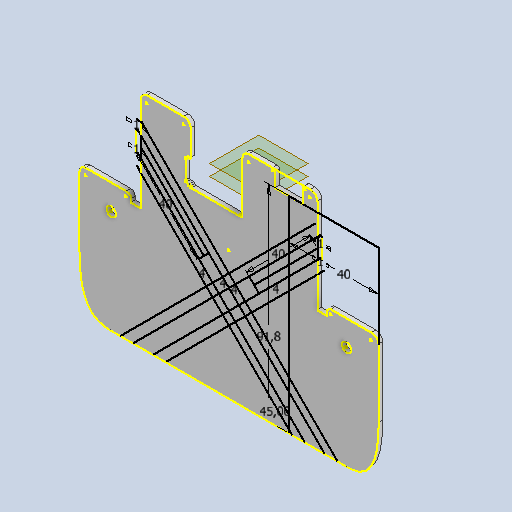
# Autodesk Inventor part: commutationCATboard
Saved by Autodesk Inventor 2022 (Build 260153000, 153)
## iProperties
Created: 2024-07-28
Part Number: commutationCATboard
Material: Типовые
Document SubType Name: Modeling
Designer: Капустяник Андрей
Density: 1 g/cm^3
Appearance: По умолчанию
Author: Капустяник Андрей
Autodesk Inventor part; units mm, degrees
ref_plane "YZ Plane" through (0, 0, 0) normal (1, 0, 0) x (0, 1, 0)
ref_plane "XZ Plane" through (0, 0, 0) normal (0, 1, 0) x (-1, 0, 0)
ref_plane "XY Plane" through (0, 0, 0) normal (0, 0, 1) x (1, 0, 0)
sketch "Эскиз1" plane through (0, 0, 0) normal (0, 0, 1) x (1, 0, 0)
  line L0 (40.5, 52.5) -> (-40.5, 52.5)
  line L1 (-40.5, 52.5) -> (-40.5, -52.5)
  line L2 (-40.5, -52.5) -> (40.5, -52.5)
  line L3 (40.5, -52.5) -> (40.5, 52.5)
  line L4 (40.5, 52.5) -> (-40.5, -52.5) construction
  line L5 (-40.5, 52.5) -> (40.5, -52.5) construction
  line L6 (-14, 32.35) -> (-14, 10.65) projected
  line L7 (-19.5, 32.35) -> (-14, 32.35) projected
  line L8 (-19.5, 10.65) -> (-19.5, 32.35) projected
  line L9 (-14, 10.65) -> (-19.5, 10.65) projected
  line L10 (43.5, -38.5) -> (43.5, -0.445) projected
  line L11 (43.5, 81.5) -> (62.7947, 81.5) projected
  line L12 (62.7947, 81.5) -> (62.7947, -38.5) projected
  line L13 (62.7947, -38.5) -> (43.5, -38.5) projected
  line L14 (-43.5, 81.5) -> (-43.5, 44.5704) projected
  line L15 (-43.5, -38.5) -> (-62.7947, -38.5) projected
  line L16 (-62.7947, -38.5) -> (-62.7947, 81.5) projected
  line L17 (-62.7947, 81.5) -> (-43.5, 81.5) projected
  line L18 (5, 81.5) -> (-5, 81.5) projected
  line L19 (-5, 81.5) -> (-5, 100.5) projected
  line L20 (-5, 100.5) -> (-52.7636, 100.5) projected
  spline S0 degree 4 poles (-64.1096, 93.28) (-61.9791, 96.5946) (-57.9302, 99.8171) (-55.7161, 100.5) (-52.7636, 100.5) knots 0 0 0 0 0 1 1 1 1 1 projected
  spline S1 degree 2 poles (-66.7947, 76.5) (-67.1982, 88.4748) (-64.1096, 93.28) knots 0 0 0 0.595731 0.595731 0.595731 projected
  line L21 (-66.7947, -33.5) -> (-66.7947, 76.5) projected
  spline S2 degree 2 poles (-66.7947, -33.5) (-67.1982, -45.4748) (-64.1096, -50.28) knots 0 0 0 0.595731 0.595731 0.595731 projected
  spline S3 degree 4 poles (-64.1096, -50.28) (-64.1007, -50.2939) (-64.0918, -50.3077) (-64.0828, -50.3215) (-64.0738, -50.3354) knots 0 0 0 0 0 0.004174 0.004174 0.004174 0.004174 0.004174 projected
  spline S4 degree 4 poles (-63.2279, -51.5022) (-63.4539, -51.2466) (-63.6704, -50.967) (-63.8771, -50.6631) (-64.0738, -50.3354) knots -0.674888 -0.674888 -0.674888 -0.674888 -0.674888 -0.60128 -0.60128 -0.60128 -0.60128 -0.60128 projected
  spline S5 degree 4 poles (-63.2279, -51.5022) (-60.8937, -54.4302) (-57.5114, -56.9383) (-55.4411, -57.5) (-52.7636, -57.5) knots 0.093114 0.093114 0.093114 0.093114 0.093114 1 1 1 1 1 projected
  line L22 (-6, -57.5) -> (-52.7636, -57.5) projected
  line L23 (-6, -57.5) -> (-6, -41.6467) projected
  arc A0 (-5, -40.6467) -> (-6, -41.6467) centre (-5, -41.6467) ccw projected
  line L24 (-5, -40.6467) -> (5, -40.6467) projected
  arc A1 (6, -41.6467) -> (5, -40.6467) centre (5, -41.6467) ccw projected
  line L25 (6, -41.6467) -> (6, -57.5) projected
  line L26 (52.7636, -57.5) -> (6, -57.5) projected
  spline S6 degree 4 poles (64.1096, -50.28) (61.9791, -53.5946) (57.9302, -56.8171) (55.7161, -57.5) (52.7636, -57.5) knots 0 0 0 0 0 1 1 1 1 1 projected
  spline S7 degree 2 poles (66.7947, -33.5) (67.1982, -45.4748) (64.1096, -50.28) knots 0 0 0 0.595731 0.595731 0.595731 projected
  line L27 (66.7947, 76.5) -> (66.7947, -33.5) projected
  spline S8 degree 2 poles (64.1096, 93.28) (67.1982, 88.4748) (66.7947, 76.5) knots -0.595731 -0.595731 -0.595731 0 0 0 projected
  spline S9 degree 4 poles (64.1096, 93.28) (61.9791, 96.5946) (57.9302, 99.8171) (55.7161, 100.5) (52.7636, 100.5) knots 0 0 0 0 0 1 1 1 1 1 projected
  line L28 (52.7636, 100.5) -> (5, 100.5) projected
  line L29 (5, 100.5) -> (5, 81.5) projected
  line L30 (33.1, -39.1) -> (40.1, -39.1) projected
  line L31 (40.1, -39.1) -> (40.1, -53.2) projected
  line L32 (40.1, -53.2) -> (33.1, -53.2) projected
  line L33 (33.1, -53.2) -> (33.1, -39.1) projected
  line L34 (-40.1, -39.25) -> (-33.1, -39.25) projected
  line L35 (-33.1, -39.25) -> (-33.1, -53.2) projected
  line L36 (-33.1, -53.2) -> (-40.1, -53.2) projected
  line L37 (-40.1, -53.2) -> (-40.1, -39.25) projected
  line L38 (-3.8, 71.4698) -> (15.7, 71.4698) projected
  arc A2 (18.7, 68.4698) -> (15.7, 71.4698) centre (15.7, 68.4698) ccw projected
  line L39 (18.7, 68.4698) -> (18.7, 55.2061) projected
  arc A3 (15.7, 52.2061) -> (18.7, 55.2061) centre (15.7, 55.2061) ccw projected
  line L40 (15.7, 52.2061) -> (-3.8, 52.2061) projected
  arc A4 (-6.8, 55.2061) -> (-3.8, 52.2061) centre (-3.8, 55.2061) ccw projected
  line L41 (-6.8, 55.2061) -> (-6.8, 68.4698) projected
  arc A5 (-3.8, 71.4698) -> (-6.8, 68.4698) centre (-3.8, 68.4698) ccw projected
  line L42 (40.5, -14.6467) -> (40.5, -35.25) projected
  line L43 (40.5, -35.25) -> (25.5, -35.25) projected
  line L44 (27.6138, 43.5704) -> (40, 43.5704) projected
  line L45 (-27.6138, 43.5704) -> (-27.6138, 44.6963) projected
  line L46 (-27.6138, 44.6963) -> (-10.238, 44.6963) projected
  line L47 (-10.238, 44.6963) -> (-10.238, 43.5704) projected
  line L48 (-10.238, 43.5704) -> (-5, 43.5704) projected
  line L49 (-5, 43.5704) -> (-5, 46.5704) projected
  line L50 (-5, 46.5704) -> (5, 46.5704) projected
  line L51 (5, 46.5704) -> (5, 43.5704) projected
  line L52 (10.238, 43.5704) -> (10.238, 44.6963) projected
  line L53 (10.238, 44.6963) -> (27.6138, 44.6963) projected
  line L54 (27.6138, 44.6963) -> (27.6138, 43.5704) projected
  line L55 (5, 43.5704) -> (10.238, 43.5704) projected
  line L56 (-43.5, 41.5) -> (43.5, 41.5)
  line L57 (43.5, 41.5) -> (43.5, -57.5)
  line L58 (43.5, -57.5) -> (-43.5, -57.5)
  line L59 (-43.5, -57.5) -> (-43.5, 41.5)
  line L60 (40, 41.5) -> (-40, 41.5) projected
  line L61 (25.5, -35.25) -> (25.5, -14.6467) projected
  line L62 (25.5, -14.6467) -> (40.5, -14.6467) projected
  line L63 (-40, 43.5704) -> (-27.6138, 43.5704) projected
  line L64 (43.5, 44.5704) -> (43.5, 81.5) projected
  line L65 (43.5, -0.445) -> (-43.5, -0.445) projected
  line L66 (-43.5, -0.445) -> (-43.5, -38.5) projected
  line L67 (40, 44.5704) -> (43.5, 44.5704) projected
  line L68 (-43.5, 44.5704) -> (-40, 44.5704) projected
  line L69 (-40, 44.5704) -> (-40, 43.5704) projected
  line L70 (40, 43.5704) -> (40, 44.5704) projected
  circle A6 centre (33.954, 52.6704) radius 1.5 projected
  circle A7 centre (23.0046, 73.1714) radius 1.5 projected
  circle A8 centre (-23.0046, 73.1714) radius 1.5 projected
  circle A9 centre (-33.954, 52.6704) radius 1.5 projected
  circle A10 centre (35.5, -5.945) radius 1.25 projected
  circle A11 centre (-35.5, -5.945) radius 1.25 projected
  point P0 (0, 0)
  point P1 (-40.5, 41.35)
  point P2 (40.5, 41.35)
  point P3 (40.5, 43.5704)
  point P4 (-40.5, -35.25)
  point P5 (-40.5, 43.5704)
  point P6 (-40.5, 41.5)
  point P7 (43.5, 41.5)
  point P8 (40.5, 41.5)
  point P9 (40.5, -0.445)
  point P10 (-40.5, -0.445)
  dimension "d0" = 81
  dimension "d1" = 105
  constraints: 20 end point, 4 parallel, 4 point on line, 2 collinear, 2 horizontal, 2 midpoint, 2 perpendicular
  measures "d0" distance of L2.end L1.end
  measures "d1" distance of L1.end L0.end
extrude "Выдавливание1" add sketch "Эскиз1" along normal blind 2 contours L56 L57 L65 L3 | L3 L65 L1 L56 | L65 L10 L57 L26 L25 L2 L33 L32 L31 L3 | L3 L62 L61 L43 L2 L31 L30 L33 L25 A1 L24 A0 L23 L35 L34 L37 L1 L65 | L3 L43 L61 L62 | L65 L59 L56 L1 | L1 L2 L37 L36 L35 L23 L22 L59 L65 | L37 L34 L35 L2 | L2 L35 L36 L37 | L31 L32 L33 L2 | L2 L33 L30 L31 | L58 L23 L2 L25 | L2 L23 A0 L24 A1 L25 | L6 L9 L8 L7 | A10 | A11
ref_plane "РабПлоскость2" through (0, 21.5, -11.5) normal (0, -1, 0) x (0, 0, 1)
sketch "Эскиз3" plane through (0, 21.5, -11.5) normal (0, -1, 0) x (0, 0, 1)
  circle A0 centre (55, 0) radius 45.02 projected
  circle A1 centre (55, 0) radius 44.1511 projected
  line L0 (13.5, -40.5) -> (13.5, 40.5) projected
  line L1 (11.5, -40.5) -> (11.5, 40.5) projected
  line L2 (13.5, 17.4514) -> (13.5, 19.4514)
  line L3 (13.5, 19.4514) -> (11.5, 19.4514)
  line L4 (13.5, -17.4514) -> (13.5, -19.4514)
  line L5 (13.5, -19.4514) -> (11.5, -19.4514)
  line L6 (11.5, -19.4514) -> (11.5, 19.4514)
  line L7 (16, 22.49) -> (55, 0) projected
  line L8 (55, 0) -> (10.66, 7.7949) projected
  line L9 (55, 0) -> (11.0199, 3.882) projected
  line L10 (15, 18.69) -> (55, 0) projected
  line L11 (16, 22.49) -> (15, 18.69)
  line L12 (10.66, 7.7949) -> (11.0199, 3.882)
  line L13 (15, 18.69) -> (15, 1.69) projected
  line L14 (11.0199, 3.882) -> (15.339, -7.9675)
  line L15 (13.5, -2.9221) -> (13.5, -5.9221)
  line L16 (13.5, -5.9221) -> (11.5, -5.9221)
  point P0 (11.5, 0)
  dimension "d5" = 2
  dimension "d6" = 2
  dimension "d15" = 165.23
  dimension "d16" = 3
  constraints: 20 end point, 10 point on line, 3 perpendicular, 3 point on circle, 1 collinear
  measures "d5" distance of L2.start L2.end
  measures "d6" distance of L4.start L4.end
  measures "d15" angle of L12 L14
  measures "d16" distance of L15.start L15.end
extrude "Выдавливание2" cut sketch "Эскиз3" along normal mid plane 10 contours L0 A1 L8 L1 A0 | A0 L1 L3 L0 | L0 L8 A1 | L16 L1 L14 L0 | L8 A1 L1 | L8 L0 L9 L1 A1 | L14 L1 L9 L0
ref_plane "РабПлоскость3" through (0, 26.5, -11.5) normal (0, -1, 0) x (1, 0, 0)
sketch "Эскиз4" plane through (0, 26.5, -11.5) normal (0, -1, 0) x (1, 0, 0)
  circle A0 centre (0, 55) radius 44.1511 projected
  line L0 (5.9221, 11.5) -> (-19.4514, 11.5) projected
  line L1 (-19.4514, 13.5) -> (5.9221, 13.5) projected
  line L2 (-19.4514, 11.5) -> (-19.4514, 13.5) projected
  line L3 (-19.4514, 13.5) -> (5.9221, 13.5) projected
  line L4 (-15.0687, 13.5) -> (-17.0687, 13.5)
  line L5 (-17.0687, 13.5) -> (-17.0687, 11.5)
  line L6 (5.9221, 11.5) -> (-19.4514, 11.5) projected
  line L7 (15.0687, 13.5) -> (17.0687, 13.5)
  line L8 (17.0687, 13.5) -> (17.0687, 11.5)
  line L9 (5.9221, 13.5) -> (5.9221, 11.5) projected
  point P0 (0, 11.5)
  point P1 (19.4514, 11.5)
  point P2 (19.4514, 13.5)
  dimension "d9" = 2
  dimension "d10" = 2
  constraints: 8 end point, 6 point on line, 2 perpendicular, 2 point on circle
  measures "d9" distance of L4.start L4.end
  measures "d10" distance of L7.start L7.end
extrude "Выдавливание3" cut sketch "Эскиз4" along normal blind 11 and the other way blind 16 contours L1 L9 L0 A0 | A0 L0 L5 L1 picked at (1.4299, 12.1667)
sketch "Эскиз5" plane through (0, 0, 2) normal (0, 0, 1) x (1, 0, 0)
  spline S0 degree 4 poles (40.5, -53.0618) (41.2011, -53.0618) (41.9466, -53.063) (42.7177, -53.0609) (43.5, -53.0523) knots -1 -1 -1 -1 -1 -0.915563 -0.915563 -0.915563 -0.915563 -0.915563 projected
  line L0 (43.5, -53.0523) -> (43.5, 100.5) projected
  line L1 (40.5, 100.5) -> (43.5, 100.5) projected
  line L2 (40.5, 100.5) -> (40.5, -53.0618) projected
  spline S1 degree 4 poles (-40.5, 96.0618) (-41.2011, 96.0618) (-41.9466, 96.063) (-42.7177, 96.0609) (-43.5, 96.0523) knots -1 -1 -1 -1 -1 -0.915563 -0.915563 -0.915563 -0.915563 -0.915563 projected
  line L3 (-43.5, 96.0523) -> (-43.5, -57.5) projected
  line L4 (-40.5, -57.5) -> (-43.5, -57.5) projected
  line L5 (-40.5, -57.5) -> (-40.5, 96.0618) projected
  line L6 (-40, 43.5704) -> (-27.6138, 43.5704) projected
  line L7 (43.5, -38.5) -> (43.5, -0.445) projected
  line L8 (43.5, 81.5) -> (62.7947, 81.5) projected
  line L9 (62.7947, 81.5) -> (62.7947, -38.5) projected
  line L10 (62.7947, -38.5) -> (43.5, -38.5) projected
  line L11 (43.5, -0.445) -> (-43.5, -0.445) projected
  line L12 (-43.5, -0.445) -> (-43.5, -38.5) projected
  line L13 (-43.5, -38.5) -> (-62.7947, -38.5) projected
  line L14 (-62.7947, -38.5) -> (-62.7947, 81.5) projected
  line L15 (-62.7947, 81.5) -> (-43.5, 81.5) projected
  line L16 (-43.5, 81.5) -> (-43.5, 44.5704) projected
  line L17 (5, 43.5704) -> (10.238, 43.5704) projected
  line L18 (-27.6138, 43.5704) -> (-27.6138, 44.6963) projected
  line L19 (-27.6138, 44.6963) -> (-10.238, 44.6963) projected
  line L20 (-10.238, 44.6963) -> (-10.238, 43.5704) projected
  line L21 (-10.238, 43.5704) -> (-5, 43.5704) projected
  line L22 (-5, 43.5704) -> (-5, 46.5704) projected
  line L23 (-5, 46.5704) -> (5, 46.5704) projected
  line L24 (5, 46.5704) -> (5, 43.5704) projected
  line L25 (10.238, 43.5704) -> (10.238, 44.6963) projected
  line L26 (10.238, 44.6963) -> (27.6138, 44.6963) projected
  line L27 (27.6138, 44.6963) -> (27.6138, 43.5704) projected
  line L28 (40.5, -14.6467) -> (40.5, -35.25) projected
  line L29 (40.5, -35.25) -> (25.5, -35.25) projected
  line L30 (25.5, -35.25) -> (25.5, -14.6467) projected
  line L31 (25.5, -14.6467) -> (40.5, -14.6467) projected
  circle A0 centre (35.9351, 52.8204) radius 2.1 projected
  circle A1 centre (23.0037, 73.1987) radius 2.1 projected
  circle A2 centre (-23.0037, 73.1987) radius 2.1 projected
  circle A3 centre (-35.954, 52.8204) radius 2.1 projected
  line L32 (5, 81.5) -> (-5, 81.5) projected
  line L33 (-5, 81.5) -> (-5, 100.5) projected
  line L34 (-5, 100.5) -> (-52.7636, 100.5) projected
  spline S2 degree 4 poles (-64.1101, 93.2803) (-61.9796, 96.5949) (-57.9303, 99.8172) (-55.7161, 100.5) (-52.7636, 100.5) knots 0 0 0 0 0 1 1 1 1 1 projected
  spline S3 degree 2 poles (-66.7947, 76.5) (-67.1987, 88.4751) (-64.1101, 93.2803) knots 0 0 0 0.595719 0.595719 0.595719 projected
  line L35 (-66.7947, -33.5) -> (-66.7947, 76.5) projected
  spline S4 degree 2 poles (-66.7947, -33.5) (-67.1987, -45.4751) (-64.1101, -50.2803) knots 0 0 0 0.595719 0.595719 0.595719 projected
  spline S5 degree 4 poles (-64.1101, -50.2803) (-64.0991, -50.2975) (-64.088, -50.3146) (-64.0768, -50.3318) (-64.0656, -50.349) knots 0 0 0 0 0 0.005185 0.005185 0.005185 0.005185 0.005185 projected
  spline S6 degree 4 poles (-63.2351, -51.4941) (-63.4567, -51.2426) (-63.6691, -50.968) (-63.8722, -50.67) (-64.0656, -50.349) knots -0.674306 -0.674306 -0.674306 -0.674306 -0.674306 -0.602047 -0.602047 -0.602047 -0.602047 -0.602047 projected
  spline S7 degree 4 poles (-63.2351, -51.4941) (-60.9013, -54.4251) (-57.5145, -56.9376) (-55.4431, -57.5) (-52.7636, -57.5) knots 0.092468 0.092468 0.092468 0.092468 0.092468 1 1 1 1 1 projected
  line L36 (-6, -57.5) -> (-52.7636, -57.5) projected
  line L37 (-6, -57.5) -> (-6, -41.6467) projected
  arc A4 (-5, -40.6467) -> (-6, -41.6467) centre (-5, -41.6467) ccw projected
  line L38 (-5, -40.6467) -> (5, -40.6467) projected
  arc A5 (6, -41.6467) -> (5, -40.6467) centre (5, -41.6467) ccw projected
  line L39 (6, -41.6467) -> (6, -57.5) projected
  line L40 (52.7636, -57.5) -> (6, -57.5) projected
  spline S8 degree 4 poles (64.1101, -50.2803) (61.9796, -53.5949) (57.9303, -56.8172) (55.7161, -57.5) (52.7636, -57.5) knots 0 0 0 0 0 1 1 1 1 1 projected
  spline S9 degree 2 poles (66.7947, -33.5) (67.1987, -45.4751) (64.1101, -50.2803) knots 0 0 0 0.595719 0.595719 0.595719 projected
  line L41 (66.7947, 76.5) -> (66.7947, -33.5) projected
  spline S10 degree 2 poles (64.1101, 93.2803) (67.1987, 88.4751) (66.7947, 76.5) knots -0.595719 -0.595719 -0.595719 0 0 0 projected
  spline S11 degree 4 poles (64.1101, 93.2803) (61.9796, 96.5949) (57.9303, 99.8172) (55.7161, 100.5) (52.7636, 100.5) knots 0 0 0 0 0 1 1 1 1 1 projected
  line L42 (52.7636, 100.5) -> (5, 100.5) projected
  line L43 (5, 100.5) -> (5, 81.5) projected
  line L44 (33.1, -39.1) -> (40.1, -39.1) projected
  line L45 (40.1, -39.1) -> (40.1, -53.2) projected
  line L46 (40.1, -53.2) -> (33.1, -53.2) projected
  line L47 (33.1, -53.2) -> (33.1, -39.1) projected
  line L48 (-40.1, -39.25) -> (-33.1, -39.25) projected
  line L49 (-33.1, -39.25) -> (-33.1, -53.2) projected
  line L50 (-33.1, -53.2) -> (-40.1, -53.2) projected
  line L51 (-40.1, -53.2) -> (-40.1, -39.25) projected
  line L52 (-3.8, 71.4698) -> (15.7, 71.4698) projected
  arc A6 (18.7, 68.4698) -> (15.7, 71.4698) centre (15.7, 68.4698) ccw projected
  line L53 (18.7, 68.4698) -> (18.7, 55.2061) projected
  arc A7 (15.7, 52.2061) -> (18.7, 55.2061) centre (15.7, 55.2061) ccw projected
  line L54 (15.7, 52.2061) -> (-3.8, 52.2061) projected
  arc A8 (-6.8, 55.2061) -> (-3.8, 52.2061) centre (-3.8, 55.2061) ccw projected
  line L55 (-6.8, 55.2061) -> (-6.8, 68.4698) projected
  arc A9 (-3.8, 71.4698) -> (-6.8, 68.4698) centre (-3.8, 68.4698) ccw projected
  line L56 (40.5, -0.445) -> (43.5, -0.445)
  line L57 (43.5, -0.445) -> (43.5, 43.5704)
  line L58 (43.5, 43.5704) -> (40.5, 43.5704)
  line L59 (40.5, 43.5704) -> (40.5, -0.445)
  line L60 (-43.5, -0.445) -> (-40.5, -0.445)
  line L61 (-40.5, -0.445) -> (-40.5, 43.5704)
  line L62 (-40.5, 43.5704) -> (-43.5, 43.5704)
  line L63 (-43.5, 43.5704) -> (-43.5, -0.445)
  line L64 (-39.5, 44.5704) -> (-39.5, -1.445)
  line L65 (-39.5, -1.445) -> (-44.5, -1.445)
  line L66 (-44.5, -1.445) -> (-44.5, 44.5704)
  line L67 (-44.5, 44.5704) -> (-39.5, 44.5704)
  line L68 (44.5, -1.445) -> (39.5, -1.445)
  line L69 (39.5, -1.445) -> (39.5, 44.5704)
  line L70 (39.5, 44.5704) -> (44.5, 44.5704)
  line L71 (44.5, 44.5704) -> (44.5, -1.445)
  line L72 (40, 45.0704) -> (43.5, 45.0704) projected
  line L73 (43.5, 45.0704) -> (43.5, 81.5) projected
  line L74 (-43.5, 44.5704) -> (-40, 44.5704) projected
  line L75 (-40, 44.5704) -> (-40, 43.5704) projected
  line L76 (27.6138, 43.5704) -> (40, 43.5704) projected
  line L77 (40, 43.5704) -> (40, 45.0704) projected
  line L78 (40.5, 0.81) -> (43.5, 0.81) projected
  line L79 (-43.5, 41.5) -> (-43.5, -57.5) projected
  line L80 (-43.5, 0.81) -> (-40.5, 0.81)
  line L81 (-44.5, 0.81) -> (-39.5, 0.81)
  line L82 (-39.5, 0.81) -> (-39.5, -0.19)
  line L83 (-39.5, -0.19) -> (-44.5, -0.19)
  line L84 (-44.5, -0.19) -> (-44.5, 0.81)
  line L85 (44.5, 0.81) -> (39.5, 0.81)
  line L86 (39.5, 0.81) -> (39.5, -0.19)
  line L87 (39.5, -0.19) -> (44.5, -0.19)
  line L88 (44.5, -0.19) -> (44.5, 0.81)
  point P0 (0, 0)
  dimension "d17" = 1
  dimension "d18" = 1
  dimension "d33" = 1
  dimension "d34" = 1
  constraints: 50 end point, 12 parallel, 10 point on line, 7 perpendicular, 4 horizontal, 3 collinear, 6 other
  measures "d17" distance between parallel lines of L61 L64
  measures "d18" distance between parallel lines of L56 L68
  measures "d33" distance of L81.end L82.end
  measures "d34" distance of L86.end L85.end
extrude "Выдавливание4" cut sketch "Эскиз5" against normal blind 2 contours L87 L2 L78 L0 | L0 L85 L71 L87 | L87 L69 L85 L2 | L78 L2 L58 L0 | L0 L70 L71 L85 | L85 L69 L76 L77 L70 L2 | L58 L2 L70 L0 | L83 L5 L81 L64 | L69 L70 L77 L76 | L83 L3 L80 L5 | L81 L5 L67 L75 L6 L64 | L80 L3 L62 L5 | L83 L66 L81 L3 | L6 L75 L67 L64 | L62 L3 L67 L5 | L81 L66 L67 L3
sketch "Эскиз8" plane through (0, 0, 2) normal (0, 0, 1) x (1, 0, 0)
  circle A0 centre (23.0046, 73.1714) radius 1.5 projected
  circle A1 centre (-23.0046, 73.1714) radius 1.5 projected
  line L0 (-3.8, 71.9698) -> (15.7, 71.9698) projected
  arc A2 (18.7, 68.9698) -> (15.7, 71.9698) centre (15.7, 68.9698) ccw projected
  line L1 (18.7, 68.9698) -> (18.7, 55.2061) projected
  arc A3 (15.7, 52.2061) -> (18.7, 55.2061) centre (15.7, 55.2061) ccw projected
  line L2 (15.7, 52.2061) -> (-3.8, 52.2061) projected
  arc A4 (-6.8, 55.2061) -> (-3.8, 52.2061) centre (-3.8, 55.2061) ccw projected
  line L3 (-6.8, 55.2061) -> (-6.8, 68.9698) projected
  arc A5 (-3.8, 71.9698) -> (-6.8, 68.9698) centre (-3.8, 68.9698) ccw projected
  line L4 (5, 81.5) -> (-5, 81.5) projected
  line L5 (-5, 81.5) -> (-5, 100.5) projected
  line L6 (-5, 100.5) -> (-52.7636, 100.5) projected
  spline S0 degree 4 poles (-52.7636, 100.5) (-55.4517, 100.5) (-58.1635, 100.1345) (-60.4837, 98.7746) (-62.3095, 96.5) knots 0 0 0 0 0 0.415412 0.415412 0.415412 0.415412 0.415412 projected
  spline S1 degree 4 poles (-62.3095, 96.5) (-64.879, 93.2991) (-66.4694, 88.287) (-66.7947, 81.6863) (-66.7947, 76.5) knots 0.415412 0.415412 0.415412 0.415412 0.415412 1 1 1 1 1 projected
  line L7 (-66.7947, -33.5) -> (-66.7947, 76.5) projected
  spline S2 degree 4 poles (-66.7947, -33.5) (-66.7947, -38.6863) (-66.4694, -45.287) (-64.879, -50.2991) (-62.3095, -53.5) knots 0 0 0 0 0 0.584588 0.584588 0.584588 0.584588 0.584588 projected
  spline S3 degree 4 poles (-62.3095, -53.5) (-60.4837, -55.7746) (-58.1635, -57.1345) (-55.4517, -57.5) (-52.7636, -57.5) knots 0.584588 0.584588 0.584588 0.584588 0.584588 1 1 1 1 1 projected
  line L8 (-52.7636, -57.5) -> (-6, -57.5) projected
  line L9 (-6, -57.5) -> (-6, -41.6467) projected
  arc A6 (-5, -40.6467) -> (-6, -41.6467) centre (-5, -41.6467) ccw projected
  line L10 (-5, -40.6467) -> (5, -40.6467) projected
  arc A7 (6, -41.6467) -> (5, -40.6467) centre (5, -41.6467) ccw projected
  line L11 (6, -41.6467) -> (6, -57.5) projected
  line L12 (6, -57.5) -> (52.7636, -57.5) projected
  spline S4 degree 4 poles (52.7636, -57.5) (55.4517, -57.5) (58.1635, -57.1345) (60.4837, -55.7746) (62.3095, -53.5) knots 0 0 0 0 0 0.415412 0.415412 0.415412 0.415412 0.415412 projected
  spline S5 degree 4 poles (62.3095, -53.5) (64.879, -50.2991) (66.4694, -45.287) (66.7947, -38.6863) (66.7947, -33.5) knots 0.415412 0.415412 0.415412 0.415412 0.415412 1 1 1 1 1 projected
  line L13 (66.7947, 76.5) -> (66.7947, -33.5) projected
  spline S6 degree 4 poles (66.7947, 76.5) (66.7947, 81.6863) (66.4694, 88.287) (64.879, 93.2991) (62.3095, 96.5) knots 0 0 0 0 0 0.584588 0.584588 0.584588 0.584588 0.584588 projected
  spline S7 degree 4 poles (62.3095, 96.5) (60.4837, 98.7746) (58.1635, 100.1345) (55.4517, 100.5) (52.7636, 100.5) knots 0.584588 0.584588 0.584588 0.584588 0.584588 1 1 1 1 1 projected
  line L14 (52.7636, 100.5) -> (5, 100.5) projected
  line L15 (5, 100.5) -> (5, 81.5) projected
  line L16 (28.4, -39.2) -> (28.4, -53.1) projected
  line L17 (28.4, -53.1) -> (21.6, -53.1) projected
  line L18 (21.6, -53.1) -> (21.6, -39.2) projected
  line L19 (21.6, -39.2) -> (28.4, -39.2) projected
  line L20 (-28.4, -39.2) -> (-21.6, -39.2) projected
  line L21 (-21.6, -39.2) -> (-21.6, -53.1) projected
  line L22 (-21.6, -53.1) -> (-28.4, -53.1) projected
  line L23 (-28.4, -53.1) -> (-28.4, -39.2) projected
  circle A8 centre (-25.5, 51) radius 1.25 projected
  circle A9 centre (25.5, -8) radius 1.25 projected
  circle A10 centre (-25.5, -8) radius 1.25 projected
  circle A11 centre (25.5, 51) radius 1.25 projected
  line L24 (-40.6, 43.5704) -> (-40.6, 61.1204) projected
  line L25 (-40.6, 61.1204) -> (-29.6, 61.1204) projected
  line L26 (-29.6, 61.1204) -> (-29.6, 43.5704) projected
  line L27 (-29.6, 43.5704) -> (-27.6138, 43.5704) projected
  line L28 (-27.6138, 43.5704) -> (-27.6138, 44.6963) projected
  line L29 (-27.6138, 44.6963) -> (-10.238, 44.6963) projected
  line L30 (-10.238, 44.6963) -> (-10.238, 43.5704) projected
  line L31 (-10.238, 43.5704) -> (-5, 43.5704) projected
  line L32 (-5, 43.5704) -> (-5, 46.5704) projected
  line L33 (-5, 46.5704) -> (5, 46.5704) projected
  line L34 (5, 46.5704) -> (5, 43.5704) projected
  line L35 (5, 43.5704) -> (10.238, 43.5704) projected
  line L36 (10.238, 43.5704) -> (10.238, 44.6963) projected
  line L37 (10.238, 44.6963) -> (27.6138, 44.6963) projected
  line L38 (27.6138, 44.6963) -> (27.6138, 43.5704) projected
  line L39 (27.6138, 43.5704) -> (43.5, 43.5704) projected
  line L40 (43.5, 43.5704) -> (43.5, 81.5) projected
  line L41 (43.5, 81.5) -> (62.7947, 81.5) projected
  line L42 (62.7947, 81.5) -> (62.7947, -38.5) projected
  line L43 (62.7947, -38.5) -> (43.5, -38.5) projected
  line L44 (43.5, -38.5) -> (43.5, -0.445) projected
  line L45 (43.5, -0.445) -> (-29.6, -0.445) projected
  line L46 (-29.6, -0.445) -> (-29.6, -15.445) projected
  line L47 (-29.6, -15.445) -> (-40.6, -15.445) projected
  line L48 (-40.6, -15.445) -> (-40.6, -0.445) projected
  line L49 (-40.6, -0.445) -> (-43.5, -0.445) projected
  line L50 (-43.5, -0.445) -> (-43.5, -38.5) projected
  line L51 (-43.5, -38.5) -> (-62.7947, -38.5) projected
  line L52 (-62.7947, -38.5) -> (-62.7947, 81.5) projected
  line L53 (-62.7947, 81.5) -> (-43.5, 81.5) projected
  line L54 (-43.5, 81.5) -> (-43.5, 43.5704) projected
  line L55 (-43.5, 43.5704) -> (-40.6, 43.5704) projected
  line L56 (39.5, -0.19) -> (39.5, 41.5) projected
  line L57 (39.5, 41.5) -> (5.9221, 41.5) projected
  line L58 (5.9221, 41.5) -> (5.9221, 15.5) projected
  line L59 (5.9221, 15.5) -> (-17.0687, 15.5) projected
  line L60 (-17.0687, 15.5) -> (-17.0687, 16.5) projected
  line L61 (-17.0687, 16.5) -> (-19.4514, 16.5) projected
  line L62 (-19.4514, 16.5) -> (-19.4514, 26.5) projected
  line L63 (-19.4514, 26.5) -> (-17.0687, 26.5) projected
  line L64 (-17.0687, 26.5) -> (-17.0687, 41.5) projected
  line L65 (-17.0687, 41.5) -> (-39.5, 41.5) projected
  line L66 (-39.5, 41.5) -> (-39.5, -0.19) projected
  line L67 (-39.5, -0.19) -> (-43.5, -0.19) projected
  line L68 (-43.5, -0.19) -> (-43.5, -57.5) projected
  line L69 (-43.5, -57.5) -> (43.5, -57.5) projected
  line L70 (43.5, -57.5) -> (43.5, -0.19) projected
  line L71 (43.5, -0.19) -> (39.5, -0.19) projected
  line L72 (-66.7947, -0.19) -> (66.7947, -0.19)
  line L73 (43.5, -0.19) -> (39.5, -0.19) projected
  circle A12 centre (23.0046, 73.1714) radius 1.5 projected
  circle A13 centre (-23.0046, 73.1714) radius 1.5 projected
  line L74 (-3.8, 71.9698) -> (15.7, 71.9698) projected
  arc A14 (18.7, 68.9698) -> (15.7, 71.9698) centre (15.7, 68.9698) ccw projected
  line L75 (18.7, 68.9698) -> (18.7, 55.2061) projected
  arc A15 (15.7, 52.2061) -> (18.7, 55.2061) centre (15.7, 55.2061) ccw projected
  line L76 (15.7, 52.2061) -> (-3.8, 52.2061) projected
  arc A16 (-6.8, 55.2061) -> (-3.8, 52.2061) centre (-3.8, 55.2061) ccw projected
  line L77 (-6.8, 55.2061) -> (-6.8, 68.9698) projected
  arc A17 (-3.8, 71.9698) -> (-6.8, 68.9698) centre (-3.8, 68.9698) ccw projected
  line L78 (5, 81.5) -> (-5, 81.5) projected
  line L79 (-5, 81.5) -> (-5, 100.5) projected
  line L80 (-5, 100.5) -> (-52.7636, 100.5) projected
  spline S8 degree 4 poles (-52.7636, 100.5) (-55.4517, 100.5) (-58.1635, 100.1345) (-60.4837, 98.7746) (-62.3095, 96.5) knots 0 0 0 0 0 0.415412 0.415412 0.415412 0.415412 0.415412 projected
  spline S9 degree 4 poles (-62.3095, 96.5) (-64.879, 93.2991) (-66.4694, 88.287) (-66.7947, 81.6863) (-66.7947, 76.5) knots 0.415412 0.415412 0.415412 0.415412 0.415412 1 1 1 1 1 projected
  line L81 (-66.7947, -33.5) -> (-66.7947, 76.5) projected
  spline S10 degree 4 poles (-66.7947, -33.5) (-66.7947, -38.6863) (-66.4694, -45.287) (-64.879, -50.2991) (-62.3095, -53.5) knots 0 0 0 0 0 0.584588 0.584588 0.584588 0.584588 0.584588 projected
  spline S11 degree 4 poles (-62.3095, -53.5) (-60.4837, -55.7746) (-58.1635, -57.1345) (-55.4517, -57.5) (-52.7636, -57.5) knots 0.584588 0.584588 0.584588 0.584588 0.584588 1 1 1 1 1 projected
  line L82 (-52.7636, -57.5) -> (-17.5, -57.5) projected
  line L83 (-17.5, -57.5) -> (-17.5, -46.5) projected
  line L84 (-17.5, -46.5) -> (-6, -46.5) projected
  line L85 (-6, -46.5) -> (-6, -41.6467) projected
  arc A18 (-5, -40.6467) -> (-6, -41.6467) centre (-5, -41.6467) ccw projected
  line L86 (-5, -40.6467) -> (5, -40.6467) projected
  arc A19 (6, -41.6467) -> (5, -40.6467) centre (5, -41.6467) ccw projected
  line L87 (6, -41.6467) -> (6, -46.5) projected
  line L88 (6, -46.5) -> (17.5, -46.5) projected
  line L89 (17.5, -46.5) -> (17.5, -57.5) projected
  line L90 (17.5, -57.5) -> (52.7636, -57.5) projected
  spline S12 degree 4 poles (52.7636, -57.5) (55.4517, -57.5) (58.1635, -57.1345) (60.4837, -55.7746) (62.3095, -53.5) knots 0 0 0 0 0 0.415412 0.415412 0.415412 0.415412 0.415412 projected
  spline S13 degree 4 poles (62.3095, -53.5) (64.879, -50.2991) (66.4694, -45.287) (66.7947, -38.6863) (66.7947, -33.5) knots 0.415412 0.415412 0.415412 0.415412 0.415412 1 1 1 1 1 projected
  line L91 (66.7947, 76.5) -> (66.7947, -33.5) projected
  spline S14 degree 4 poles (66.7947, 76.5) (66.7947, 81.6863) (66.4694, 88.287) (64.879, 93.2991) (62.3095, 96.5) knots 0 0 0 0 0 0.584588 0.584588 0.584588 0.584588 0.584588 projected
  spline S15 degree 4 poles (62.3095, 96.5) (60.4837, 98.7746) (58.1635, 100.1345) (55.4517, 100.5) (52.7636, 100.5) knots 0.584588 0.584588 0.584588 0.584588 0.584588 1 1 1 1 1 projected
  line L92 (52.7636, 100.5) -> (5, 100.5) projected
  line L93 (5, 100.5) -> (5, 81.5) projected
  line L94 (21.9, -38.9) -> (29.3, -38.9) projected
  line L95 (29.3, -38.9) -> (29.3, -53.4) projected
  line L96 (29.3, -53.4) -> (21.9, -53.4) projected
  line L97 (21.9, -53.4) -> (21.9, -38.9) projected
  line L98 (-29.3, -38.9) -> (-21.9, -38.9) projected
  line L99 (-21.9, -38.9) -> (-21.9, -53.4) projected
  line L100 (-21.9, -53.4) -> (-29.3, -53.4) projected
  line L101 (-29.3, -53.4) -> (-29.3, -38.9) projected
  circle A20 centre (-25.5, 51) radius 1.25 projected
  circle A21 centre (25.5, -8) radius 1.25 projected
  circle A22 centre (-25.5, -8) radius 1.25 projected
  circle A23 centre (25.5, 51) radius 1.25 projected
  line L102 (-40.6, 43.5704) -> (-40.6, 61.1204) projected
  line L103 (-40.6, 61.1204) -> (-29.6, 61.1204) projected
  line L104 (-29.6, 61.1204) -> (-29.6, 43.5704) projected
  line L105 (-29.6, 43.5704) -> (-27.6138, 43.5704) projected
  line L106 (-27.6138, 43.5704) -> (-27.6138, 44.6963) projected
  line L107 (-27.6138, 44.6963) -> (-10.238, 44.6963) projected
  line L108 (-10.238, 44.6963) -> (-10.238, 43.5704) projected
  line L109 (-10.238, 43.5704) -> (-5, 43.5704) projected
  line L110 (-5, 43.5704) -> (-5, 46.5704) projected
  line L111 (-5, 46.5704) -> (5, 46.5704) projected
  line L112 (5, 46.5704) -> (5, 43.5704) projected
  line L113 (5, 43.5704) -> (10.238, 43.5704) projected
  line L114 (10.238, 43.5704) -> (10.238, 44.6963) projected
  line L115 (10.238, 44.6963) -> (27.6138, 44.6963) projected
  line L116 (27.6138, 44.6963) -> (27.6138, 43.5704) projected
  line L117 (27.6138, 43.5704) -> (43.5, 43.5704) projected
  line L118 (43.5, 43.5704) -> (43.5, 81.5) projected
  line L119 (43.5, 81.5) -> (62.7947, 81.5) projected
  line L120 (62.7947, 81.5) -> (62.7947, -38.5) projected
  line L121 (62.7947, -38.5) -> (43.5, -38.5) projected
  line L122 (43.5, -38.5) -> (43.5, -0.445) projected
  line L123 (43.5, -0.445) -> (-29.6, -0.445) projected
  line L124 (-29.6, -0.445) -> (-29.6, -15.445) projected
  line L125 (-29.6, -15.445) -> (-40.6, -15.445) projected
  line L126 (-40.6, -15.445) -> (-40.6, -0.445) projected
  line L127 (-40.6, -0.445) -> (-43.5, -0.445) projected
  line L128 (-43.5, -0.445) -> (-43.5, -38.5) projected
  line L129 (-43.5, -38.5) -> (-62.7947, -38.5) projected
  line L130 (-62.7947, -38.5) -> (-62.7947, 81.5) projected
  line L131 (-62.7947, 81.5) -> (-43.5, 81.5) projected
  line L132 (-43.5, 81.5) -> (-43.5, 43.5704) projected
  line L133 (-43.5, 43.5704) -> (-40.6, 43.5704) projected
  point P0 (8, -57.5)
  point P1 (-8, -57.5)
  point P2 (43.5, -0.19)
  constraints: 2 end point, 2 point on line, 1 collinear, 1 perpendicular
extrude "Выдавливание7" add sketch "Эскиз8" against normal blind 2 contours L13 S5 S4 L12 L70 L43 L42 L72 | L72 L52 L51 L68 L8 S3 S2 L7 | L42 L43 L44 L70 L72 | L72 L68 L50 L51 L52
fillet "Сопряжение1" radius 3 6 edges at (-39.5, 41.5, 1) (-17.0687, 41.5, 1) (39.5, 41.5, 1) (5.9221, 41.5, 1) (-66.7947, -0.19, 1) (66.7947, -0.19, 1)
fillet "Сопряжение2" radius 0.5 6 edges at (-17.0687, 26.5, 1) (-19.4514, 26.5, 1) (-19.4514, 16.5, 1) (-17.0687, 16.5, 1) (-17.0687, 15.5, 1) (5.9221, 15.5, 1)
sketch "Эскиз9" plane through (0, 0, 2) normal (0, 0, 1) x (1, 0, 0)
  arc A0 (-17.0687, 16) -> (-17.5687, 16.5) centre (-17.5687, 16) ccw projected
  line L0 (-17.5687, 16.5) -> (-18.9514, 16.5) projected
  arc A1 (-19.4514, 17) -> (-18.9514, 16.5) centre (-18.9514, 17) ccw projected
  line L1 (-19.4514, 17) -> (-19.4514, 26) projected
  arc A2 (-18.9514, 26.5) -> (-19.4514, 26) centre (-18.9514, 26) ccw projected
  line L2 (-18.9514, 26.5) -> (-17.5687, 26.5) projected
  arc A3 (-17.5687, 26.5) -> (-17.0687, 27) centre (-17.5687, 27) ccw projected
  line L3 (-17.0687, 27) -> (-17.0687, 38.5) projected
  arc A4 (-17.0687, 38.5) -> (-20.0687, 41.5) centre (-20.0687, 38.5) ccw projected
  line L4 (-20.0687, 41.5) -> (-36.5, 41.5) projected
  arc A5 (-36.5, 41.5) -> (-39.5, 38.5) centre (-36.5, 38.5) ccw projected
  line L5 (-39.5, 38.5) -> (-39.5, -0.19) projected
  line L6 (39.5, -0.19) -> (39.5, 38.5) projected
  arc A6 (39.5, 38.5) -> (36.5, 41.5) centre (36.5, 38.5) ccw projected
  line L7 (36.5, 41.5) -> (8.9221, 41.5) projected
  line L8 (5.9221, 38.5) -> (5.9221, 16) projected
  arc A7 (5.4221, 15.5) -> (5.9221, 16) centre (5.4221, 16) ccw projected
  line L9 (5.4221, 15.5) -> (-16.5687, 15.5) projected
  arc A8 (-17.0687, 16) -> (-16.5687, 15.5) centre (-16.5687, 16) ccw projected
  line L10 (39.6, -3.445) -> (43.5, -3.445) projected
  line L11 (39.5, -0.19) -> (43.5, -0.19)
  line L12 (43.5, -0.19) -> (43.5, -3.445)
  line L13 (43.5, -3.445) -> (39.5, -3.445)
  line L14 (39.5, -3.445) -> (39.5, -0.19)
  line L15 (43.65, -3.595) -> (43.65, -0.04)
  line L16 (43.65, -0.04) -> (39.35, -0.04)
  line L17 (39.35, -0.04) -> (39.35, -3.595)
  line L18 (39.35, -3.595) -> (43.65, -3.595)
  line L19 (39.5, -0.19) -> (63.7947, -0.19) projected
  line L20 (39.5, -0.19) -> (39.5, -3.595)
  arc A9 (8.9221, 41.5) -> (5.9221, 38.5) centre (8.9221, 38.5) ccw projected
  line L21 (-39.5, -0.19) -> (-63.7947, -0.19) projected
  line L22 (63.7947, -0.19) -> (39.5, -0.19) projected
  line L23 (-66.7947, -3.19) -> (-66.7947, -33.5) projected
  line L24 (-52.7636, -57.5) -> (52.7636, -57.5) projected
  line L25 (66.7947, -33.5) -> (66.7947, -3.19) projected
  arc A10 (-63.7947, -0.19) -> (-66.7947, -3.19) centre (-63.7947, -3.19) ccw projected
  arc A11 (66.7947, -3.19) -> (63.7947, -0.19) centre (63.7947, -3.19) ccw projected
  point P0 (0, 0)
  point P1 (-62.3095, -53.5)
  point P2 (62.3095, -53.5)
  point P3 (66.7947, -0.19)
  point P4 (39.5, -0.04)
  dimension "d37" = 0.15
  constraints: 18 end point, 5 parallel, 2 perpendicular, 1 horizontal, 1 point on line, 7 other
  measures "d37" distance between parallel lines of L12 L15
extrude "Выдавливание8" cut sketch "Эскиз9" against normal blind 10 contours L6 L16 L15 L19 L11 | L11 L12 L10 L13 L14 | L19 L15 L18 L20 L13 L10 L12
fillet "Сопряжение3" radius 2 1 edges at (43.65, -0.19, 1)
mirror "Зеркальное отражение1" about plane through (0, 0, 0) normal (1, 0, 0) of "Выдавливание8", "Сопряжение3"
sketch "Эскиз11" plane through (0, 0, 2) normal (0, 0, 1) x (1, 0, 0)
  circle A0 centre (-52.5474, -11.39) radius 2 projected
  circle A1 centre (52.5474, -11.39) radius 2 projected
  circle A2 centre (52.5474, -11.39) radius 2.1
  circle A3 centre (-52.5474, -11.39) radius 2.1
  point P0 (0, 0)
  dimension "d50" = 4.2
  dimension "d51" = 4.2
  constraints: 2 centre point, 2 coincident
  measures "d50" diameter of A2
  measures "d51" diameter of A3
extrude "Выдавливание10" cut sketch "Эскиз11" against normal blind 10 contours A0 | A1 | A2 | A3
sketch "Эскиз12" plane through (0, 0, 2) normal (0, 0, 1) x (1, 0, 0)
  circle A0 centre (52.5474, -11.39) radius 2.1 projected
  circle A1 centre (-52.5474, -11.39) radius 2.1 projected
  arc A2 (-43.65, -2.19) -> (-45.65, -0.19) centre (-45.65, -2.19) ccw projected
  line L0 (-45.65, -0.19) -> (-63.7947, -0.19) projected
  arc A3 (-63.7947, -0.19) -> (-66.7947, -3.19) centre (-63.7947, -3.19) ccw projected
  line L1 (-66.7947, -3.19) -> (-66.7947, -33.5) projected
  line L2 (-52.7636, -57.5) -> (52.7636, -57.5) projected
  line L3 (66.7947, -33.5) -> (66.7947, -3.19) projected
  arc A4 (66.7947, -3.19) -> (63.7947, -0.19) centre (63.7947, -3.19) ccw projected
  line L4 (63.7947, -0.19) -> (45.65, -0.19) projected
  arc A5 (45.65, -0.19) -> (43.65, -2.19) centre (45.65, -2.19) ccw projected
  line L5 (43.65, -2.19) -> (43.65, -3.595) projected
  line L6 (43.65, -3.595) -> (39.5, -3.595) projected
  line L7 (39.5, -3.595) -> (39.5, 38.5) projected
  arc A6 (39.5, 38.5) -> (36.5, 41.5) centre (36.5, 38.5) ccw projected
  line L8 (36.5, 41.5) -> (8.9221, 41.5) projected
  arc A7 (8.9221, 41.5) -> (5.9221, 38.5) centre (8.9221, 38.5) ccw projected
  line L9 (5.9221, 38.5) -> (5.9221, 16) projected
  arc A8 (5.4221, 15.5) -> (5.9221, 16) centre (5.4221, 16) ccw projected
  line L10 (5.4221, 15.5) -> (-16.5687, 15.5) projected
  arc A9 (-17.0687, 16) -> (-16.5687, 15.5) centre (-16.5687, 16) ccw projected
  arc A10 (-17.0687, 16) -> (-17.5687, 16.5) centre (-17.5687, 16) ccw projected
  line L11 (-17.5687, 16.5) -> (-18.9514, 16.5) projected
  arc A11 (-19.4514, 17) -> (-18.9514, 16.5) centre (-18.9514, 17) ccw projected
  line L12 (-19.4514, 17) -> (-19.4514, 26) projected
  arc A12 (-18.9514, 26.5) -> (-19.4514, 26) centre (-18.9514, 26) ccw projected
  line L13 (-18.9514, 26.5) -> (-17.5687, 26.5) projected
  arc A13 (-17.5687, 26.5) -> (-17.0687, 27) centre (-17.5687, 27) ccw projected
  line L14 (-17.0687, 27) -> (-17.0687, 38.5) projected
  arc A14 (-17.0687, 38.5) -> (-20.0687, 41.5) centre (-20.0687, 38.5) ccw projected
  line L15 (-20.0687, 41.5) -> (-36.5, 41.5) projected
  arc A15 (-36.5, 41.5) -> (-39.5, 38.5) centre (-36.5, 38.5) ccw projected
  line L16 (-39.5, 38.5) -> (-39.5, -3.595) projected
  line L17 (-39.5, -3.595) -> (-43.65, -3.595) projected
  line L18 (-43.65, -3.595) -> (-43.65, -2.19) projected
  line L19 (41.5904, 17.05) -> (41.5904, 25.95) projected
  line L20 (-41.5904, 25.95) -> (-41.5904, 17.05) projected
  line L21 (-41.5904, 25.95) -> (-41.5904, 17.05) projected
  line L22 (-41.5904, 25.95) -> (-40.5904, 25.95)
  line L23 (-39.5, -3.595) -> (-39.5, 38.5) projected
  line L24 (-40.5904, 25.95) -> (42.8596, -57.5)
  line L25 (52.7636, -57.5) -> (-52.7636, -57.5) projected
  line L26 (-41.5904, 17.05) -> (-40.5904, 17.05)
  line L27 (-40.5904, 17.05) -> (33.9596, -57.5)
  line L28 (41.5904, 25.95) -> (40.5904, 25.95)
  line L29 (39.5, 38.5) -> (39.5, -3.595) projected
  line L30 (40.5904, 25.95) -> (-42.8596, -57.5)
  line L31 (41.5904, 17.05) -> (40.5904, 17.05)
  line L32 (40.5904, 17.05) -> (-33.9596, -57.5)
  line L33 (48.5165, -57.5) -> (-38.9335, 29.95)
  line L34 (-38.9335, 29.95) -> (-41.5904, 29.95)
  line L35 (28.3028, -57.5) -> (-41.2581, 12.0609)
  line L36 (-48.5165, -57.5) -> (38.9335, 29.95)
  line L37 (42.2472, 13.05) -> (-28.3028, -57.5)
  line L38 (39.5, 20.4096) -> (11.2157, -7.8746)
  line L39 (39.5, 24.8596) -> (39.5, 15.9596)
  line L40 (-39.5, 38.5) -> (-39.5, -3.595) projected
  line L41 (-39.5, 24.8596) -> (-39.5, 15.9596)
  line L42 (-39.5, 20.4096) -> (-11.2157, -7.8746)
  line L43 (-13.4407, -10.0996) -> (-8.9907, -5.6496)
  line L44 (8.9907, -5.6496) -> (13.4407, -10.0996)
  point P0 (0, 0)
  point P1 (-62.3095, -53.5)
  point P2 (62.3095, -53.5)
  dimension "d54" = 1
  dimension "d55" = 1
  dimension "d56" = 1
  dimension "d57" = 1
  dimension "d58" = 45
  dimension "d59" = 4
  dimension "d60" = 4
  dimension "d61" = 4
  dimension "d62" = 4
  dimension "d63" = 40
  dimension "d64" = 40
  constraints: 38 end point, 14 point on line, 5 parallel, 5 perpendicular, 4 midpoint, 1 horizontal, 14 other
  measures "d54" distance of L20.start L22.end
  measures "d55" distance of L20.end L26.end
  measures "d56" distance of L19.end L28.end
  measures "d57" distance of L19.start L31.end
  measures "d58" angle of L2 L27
  measures "d59" distance between parallel lines of L24 L33
  measures "d60" distance between parallel lines of L27 L35
  measures "d61" distance between parallel lines of L30 L36
  measures "d62" distance between parallel lines of L32 L37
  measures "d63" distance of L38.start L38.end
  measures "d64" distance of L42.start L42.end
sketch "Эскиз13" plane through (0, 0, 2) normal (0, 0, 1) x (1, 0, 0)
  circle A0 centre (52.5474, -11.39) radius 2.1 projected
  circle A1 centre (-52.5474, -11.39) radius 2.1 projected
  arc A2 (-43.65, -2.19) -> (-45.65, -0.19) centre (-45.65, -2.19) ccw projected
  line L0 (-45.65, -0.19) -> (-63.7947, -0.19) projected
  arc A3 (-63.7947, -0.19) -> (-66.7947, -3.19) centre (-63.7947, -3.19) ccw projected
  line L1 (-66.7947, -3.19) -> (-66.7947, -33.5) projected
  line L2 (-52.7636, -57.5) -> (52.7636, -57.5) projected
  line L3 (66.7947, -33.5) -> (66.7947, -3.19) projected
  arc A4 (66.7947, -3.19) -> (63.7947, -0.19) centre (63.7947, -3.19) ccw projected
  line L4 (63.7947, -0.19) -> (45.65, -0.19) projected
  arc A5 (45.65, -0.19) -> (43.65, -2.19) centre (45.65, -2.19) ccw projected
  line L5 (43.65, -2.19) -> (43.65, -3.595) projected
  line L6 (43.65, -3.595) -> (39.5, -3.595) projected
  line L7 (39.5, -3.595) -> (39.5, 38.5) projected
  arc A6 (39.5, 38.5) -> (36.5, 41.5) centre (36.5, 38.5) ccw projected
  line L8 (36.5, 41.5) -> (8.9221, 41.5) projected
  arc A7 (8.9221, 41.5) -> (5.9221, 38.5) centre (8.9221, 38.5) ccw projected
  line L9 (5.9221, 38.5) -> (5.9221, 16) projected
  arc A8 (5.4221, 15.5) -> (5.9221, 16) centre (5.4221, 16) ccw projected
  line L10 (5.4221, 15.5) -> (-16.5687, 15.5) projected
  arc A9 (-17.0687, 16) -> (-16.5687, 15.5) centre (-16.5687, 16) ccw projected
  arc A10 (-17.0687, 16) -> (-17.5687, 16.5) centre (-17.5687, 16) ccw projected
  line L11 (-17.5687, 16.5) -> (-18.9514, 16.5) projected
  arc A11 (-19.4514, 17) -> (-18.9514, 16.5) centre (-18.9514, 17) ccw projected
  line L12 (-19.4514, 17) -> (-19.4514, 26) projected
  arc A12 (-18.9514, 26.5) -> (-19.4514, 26) centre (-18.9514, 26) ccw projected
  line L13 (-18.9514, 26.5) -> (-17.5687, 26.5) projected
  arc A13 (-17.5687, 26.5) -> (-17.0687, 27) centre (-17.5687, 27) ccw projected
  line L14 (-17.0687, 27) -> (-17.0687, 38.5) projected
  arc A14 (-17.0687, 38.5) -> (-20.0687, 41.5) centre (-20.0687, 38.5) ccw projected
  line L15 (-20.0687, 41.5) -> (-36.5, 41.5) projected
  arc A15 (-36.5, 41.5) -> (-39.5, 38.5) centre (-36.5, 38.5) ccw projected
  line L16 (-39.5, 38.5) -> (-39.5, -3.595) projected
  line L17 (-39.5, -3.595) -> (-43.65, -3.595) projected
  line L18 (-43.65, -3.595) -> (-43.65, -2.19) projected
  line L19 (26.7947, 34.3) -> (66.7947, 34.3)
  line L20 (66.7947, -33.5) -> (66.7947, -3.19) projected
  line L21 (66.7947, 34.3) -> (66.7947, -3.19)
  line L22 (26.7947, 34.3) -> (26.7947, -57.5)
  line L23 (-52.7636, -57.5) -> (52.7636, -57.5) projected
  point P0 (0, 0)
  point P1 (-62.3095, -53.5)
  point P2 (62.3095, -53.5)
  dimension "d65" = 40
  dimension "d66" = 91.8
  constraints: 6 end point, 1 collinear, 1 horizontal, 1 point on line, 1 vertical, 4 other
  measures "d65" distance of L19.start L19.end
  measures "d66" distance of L19.start L22.end
sketch "Эскиз14" plane through (0, 0, 2) normal (0, 0, 1) x (1, 0, 0)
  line L0 (31.4447, 34.9) -> (30.8947, 34.9) projected
  line L1 (31.4447, 34.3) -> (31.4447, 34.9) projected
  line L2 (32.0947, 34.3) -> (31.4447, 34.3) projected
  line L3 (32.0947, 34.3) -> (32.0947, 34.9) projected
  line L4 (32.6697, 34.9) -> (32.0947, 34.9) projected
  line L5 (32.6697, 34.9) -> (32.6697, 38.5) projected
  line L6 (32.6697, 38.5) -> (20.9197, 38.5) projected
  line L7 (20.9197, 34.9) -> (20.9197, 38.5) projected
  line L8 (20.9197, 34.9) -> (21.4947, 34.9) projected
  line L9 (21.4947, 34.3) -> (21.4947, 34.9) projected
  line L10 (22.1447, 34.3) -> (21.4947, 34.3) projected
  line L11 (22.1447, 34.3) -> (22.1447, 34.9) projected
  line L12 (22.6947, 34.9) -> (22.1447, 34.9) projected
  line L13 (22.6947, 34.3) -> (22.6947, 34.9) projected
  line L14 (23.3947, 34.3) -> (22.6947, 34.3) projected
  line L15 (23.3947, 34.3) -> (23.3947, 34.9) projected
  line L16 (23.9447, 34.9) -> (23.3947, 34.9) projected
  line L17 (23.9447, 34.3) -> (23.9447, 34.9) projected
  line L18 (24.6447, 34.3) -> (23.9447, 34.3) projected
  line L19 (24.6447, 34.3) -> (24.6447, 34.9) projected
  line L20 (25.1947, 34.9) -> (24.6447, 34.9) projected
  line L21 (25.1947, 34.3) -> (25.1947, 34.9) projected
  line L22 (25.8947, 34.3) -> (25.1947, 34.3) projected
  line L23 (25.8947, 34.3) -> (25.8947, 34.9) projected
  line L24 (26.4447, 34.9) -> (25.8947, 34.9) projected
  line L25 (26.4447, 34.3) -> (26.4447, 34.9) projected
  line L26 (27.1447, 34.3) -> (26.4447, 34.3) projected
  line L27 (27.1447, 34.3) -> (27.1447, 34.9) projected
  line L28 (27.6947, 34.9) -> (27.1447, 34.9) projected
  line L29 (27.6947, 34.3) -> (27.6947, 34.9) projected
  line L30 (28.3947, 34.3) -> (27.6947, 34.3) projected
  line L31 (28.3947, 34.3) -> (28.3947, 34.9) projected
  line L32 (28.9447, 34.9) -> (28.3947, 34.9) projected
  line L33 (28.9447, 34.3) -> (28.9447, 34.9) projected
  line L34 (29.6447, 34.3) -> (28.9447, 34.3) projected
  line L35 (29.6447, 34.3) -> (29.6447, 34.9) projected
  line L36 (30.1947, 34.9) -> (29.6447, 34.9) projected
  line L37 (30.1947, 34.3) -> (30.1947, 34.9) projected
  line L38 (30.8947, 34.3) -> (30.1947, 34.3) projected
  line L39 (30.8947, 34.3) -> (30.8947, 34.9) projected
  line L40 (23.5947, 37.05) -> (22.4947, 37.05) projected
  line L41 (23.5947, 37.05) -> (23.5947, 35.9) projected
  line L42 (22.4947, 35.9) -> (23.5947, 35.9) projected
  line L43 (22.4947, 37.05) -> (22.4947, 35.9) projected
  line L44 (31.0947, 37.05) -> (29.9947, 37.05) projected
  line L45 (31.0947, 37.05) -> (31.0947, 35.9) projected
  line L46 (29.9947, 35.9) -> (31.0947, 35.9) projected
  line L47 (29.9947, 37.05) -> (29.9947, 35.9) projected
  line L48 (36.5, 41.5) -> (8.9221, 41.5) projected
  line L49 (20.6697, 34.25) -> (32.9197, 34.25)
  line L50 (32.9197, 34.25) -> (32.9197, 41.5)
  line L51 (32.9197, 41.5) -> (20.6697, 41.5)
  line L52 (20.6697, 41.5) -> (20.6697, 34.25)
  point P0 (0, 0)
  dimension "d67" = 0.25
  dimension "d68" = 0.25
  dimension "d69" = 0.05
  constraints: 8 end point, 2 parallel, 1 horizontal, 1 perpendicular, 1 point on line
  measures "d67" distance between parallel lines of L7 L52
  measures "d68" distance between parallel lines of L50 L5
  measures "d69" distance between parallel lines of L10 L49
extrude "Выдавливание11" cut sketch "Эскиз14" against normal blind 10 contours L0 L39 L38 L37 L36 L35 L34 L33 L32 L31 L30 L29 L28 L27 L26 L25 L24 L23 L22 L21 L20 L19 L18 L17 L16 L15 L14 L13 L12 L11 L10 L9 L8 L7 L6 L5 L4 L3 L2 L1 | L41 L42 L43 L40 | L45 L46 L47 L44 | L50 L49 L52 L48
fillet "Сопряжение5" radius 1 2 edges at (20.6697, 41.5, 1) (32.9197, 41.5, 1)
sketch "Эскиз15" plane through (0, 0, 2) normal (0, 0, 1) x (1, 0, 0)
  arc A0 (33.9197, 41.5) -> (32.9197, 40.5) centre (33.9197, 40.5) ccw projected
  line L0 (32.9197, 40.5) -> (32.9197, 34.25) projected
  line L1 (32.9197, 34.25) -> (20.6697, 34.25) projected
  line L2 (20.6697, 34.25) -> (20.6697, 40.5) projected
  arc A1 (20.6697, 40.5) -> (19.6697, 41.5) centre (19.6697, 40.5) ccw projected
  line L3 (19.6697, 41.5) -> (8.9221, 41.5) projected
  arc A2 (8.9221, 41.5) -> (5.9221, 38.5) centre (8.9221, 38.5) ccw projected
  line L4 (5.9221, 38.5) -> (5.9221, 16) projected
  arc A3 (5.4221, 15.5) -> (5.9221, 16) centre (5.4221, 16) ccw projected
  line L5 (5.4221, 15.5) -> (-16.5687, 15.5) projected
  arc A4 (-17.0687, 16) -> (-16.5687, 15.5) centre (-16.5687, 16) ccw projected
  arc A5 (-17.0687, 16) -> (-17.5687, 16.5) centre (-17.5687, 16) ccw projected
  line L6 (-17.5687, 16.5) -> (-18.9514, 16.5) projected
  arc A6 (-19.4514, 17) -> (-18.9514, 16.5) centre (-18.9514, 17) ccw projected
  line L7 (-19.4514, 17) -> (-19.4514, 26) projected
  arc A7 (-18.9514, 26.5) -> (-19.4514, 26) centre (-18.9514, 26) ccw projected
  line L8 (-18.9514, 26.5) -> (-17.5687, 26.5) projected
  arc A8 (-17.5687, 26.5) -> (-17.0687, 27) centre (-17.5687, 27) ccw projected
  line L9 (-17.0687, 27) -> (-17.0687, 38.5) projected
  arc A9 (-17.0687, 38.5) -> (-20.0687, 41.5) centre (-20.0687, 38.5) ccw projected
  line L10 (-20.0687, 41.5) -> (-36.5, 41.5) projected
  arc A10 (-36.5, 41.5) -> (-39.5, 38.5) centre (-36.5, 38.5) ccw projected
  line L11 (-39.5, 38.5) -> (-39.5, -3.595) projected
  line L12 (-39.5, -3.595) -> (-43.65, -3.595) projected
  line L13 (-43.65, -3.595) -> (-43.65, -2.19) projected
  arc A11 (-43.65, -2.19) -> (-45.65, -0.19) centre (-45.65, -2.19) ccw projected
  line L14 (-45.65, -0.19) -> (-63.7947, -0.19) projected
  arc A12 (-63.7947, -0.19) -> (-66.7947, -3.19) centre (-63.7947, -3.19) ccw projected
  line L15 (-66.7947, -3.19) -> (-66.7947, -33.5) projected
  line L16 (-52.7636, -57.5) -> (52.7636, -57.5) projected
  line L17 (66.7947, -33.5) -> (66.7947, -3.19) projected
  arc A13 (66.7947, -3.19) -> (63.7947, -0.19) centre (63.7947, -3.19) ccw projected
  line L18 (63.7947, -0.19) -> (45.65, -0.19) projected
  arc A14 (45.65, -0.19) -> (43.65, -2.19) centre (45.65, -2.19) ccw projected
  line L19 (43.65, -2.19) -> (43.65, -3.595) projected
  line L20 (43.65, -3.595) -> (39.5, -3.595) projected
  line L21 (39.5, -3.595) -> (39.5, 38.5) projected
  arc A15 (39.5, 38.5) -> (36.5, 41.5) centre (36.5, 38.5) ccw projected
  line L22 (36.5, 41.5) -> (33.9197, 41.5) projected
  circle A16 centre (-52.5474, -11.39) radius 2.1 projected
  circle A17 centre (52.5474, -11.39) radius 2.1 projected
  point P0 (0, 0)
  point P1 (-62.3095, -53.5)
  point P2 (62.3095, -53.5)
  constraints: 4 other
